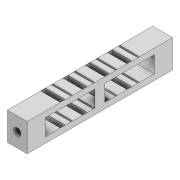
# Autodesk Inventor part: 20220727_4cell_PBME
Saved by Autodesk Inventor 2022 (Build 260153000, 153)
## iProperties
Created: 2022-07-28
Part Number: 20220727_4cell_PBME
Material: Generic
Document SubType Name: Modeling
Designer: scott
Density: 1 g/cm^3
Appearance: Default
Author: scott
Autodesk Inventor part; units mm, degrees
ref_plane "YZ Plane" through (0, 0, 0) normal (1, 0, 0) x (0, 1, 0)
ref_plane "XZ Plane" through (0, 0, 0) normal (0, 1, 0) x (-1, 0, 0)
ref_plane "XY Plane" through (0, 0, 0) normal (0, 0, 1) x (1, 0, 0)
sketch "Sketch1" plane through (0, 0, 0) normal (0, 1, 0) x (-1, 0, 0)
  line L0 (0, 0) -> (-24, 0)
  line L1 (-24, 0) -> (-24, -176.4)
  line L2 (-24, -176.4) -> (0, -176.4)
  line L3 (0, -176.4) -> (0, 0)
  dimension "d0" = 176.4
  dimension "d1" = 24
  constraints: 8 end point, 2 parallel, 1 horizontal, 1 perpendicular
  measures "d0" distance of L0.end L1.end
  measures "d1" distance of L1.end L2.end
extrude "Extrusion1" add sketch "Sketch1" along normal blind 34
sketch "Sketch2" plane through (24, 0, 0) normal (1, 0, 0) x (0, 0, -1)
  line L0 (22, 27) -> (154.4, 27)
  line L1 (154.4, 27) -> (154.4, 7)
  line L2 (154.4, 7) -> (22, 7)
  line L3 (22, 7) -> (22, 27)
  line L4 (0, 0) -> (176.4, 0) projected
  line L5 (0, 34) -> (176.4, 34) projected
  line L6 (176.4, 0) -> (176.4, 34) projected
  line L7 (0, 0) -> (0, 34) projected
  dimension "d4" = 7
  dimension "d5" = 7
  dimension "d6" = 22
  dimension "d7" = 22
  constraints: 8 end point, 2 parallel, 1 horizontal, 1 perpendicular
  measures "d4" distance between parallel lines of L4 L2
  measures "d5" distance between parallel lines of L5 L0
  measures "d6" distance between parallel lines of L6 L1
  measures "d7" distance between parallel lines of L3 L7
extrude "Extrusion2" cut sketch "Sketch2" against normal up to surface (24 mm away) contours L0 L1 L2 L3
sketch "Sketch3" plane through (0, 34, 0) normal (0, 1, 0) x (1, 0, 0)
  line L0 (0.5, 46.2) -> (23.5, 46.2)
  line L1 (23.5, 46.2) -> (23.5, 40.2)
  line L2 (23.5, 40.2) -> (0.5, 40.2)
  line L3 (0.5, 40.2) -> (0.5, 46.2)
  line L4 (0.5, 73.2) -> (23.5, 73.2)
  line L5 (23.5, 73.2) -> (23.5, 67.2)
  line L6 (23.5, 67.2) -> (0.5, 67.2)
  line L7 (0.5, 67.2) -> (0.5, 73.2)
  line L8 (0.5, 100.2) -> (23.5, 100.2)
  line L9 (23.5, 100.2) -> (23.5, 94.2)
  line L10 (23.5, 94.2) -> (0.5, 94.2)
  line L11 (0.5, 94.2) -> (0.5, 100.2)
  line L12 (0.5, 127.2) -> (23.5, 127.2)
  line L13 (23.5, 127.2) -> (23.5, 121.2)
  line L14 (23.5, 121.2) -> (0.5, 121.2)
  line L15 (0.5, 121.2) -> (0.5, 127.2)
  line L16 (0, 0) -> (24, 0) projected
  line L17 (0, 176.4) -> (0, 0) projected
  line L18 (24, 0) -> (24, 176.4) projected
  dimension "d10" = 6
  dimension "d11" = 6
  dimension "d12" = 6
  dimension "d13" = 6
  dimension "d14" = 27
  dimension "d15" = 27
  dimension "d16" = 27
  dimension "d17" = 40.2
  dimension "d18" = 0.5
  dimension "d19" = 0.5
  dimension "d20" = 0.5
  dimension "d21" = 0.5
  constraints: 32 end point, 8 parallel, 4 horizontal, 4 perpendicular, 4 point on line
  measures "d10" distance of L14.end L12.start
  measures "d11" distance of L10.end L8.start
  measures "d12" distance of L6.end L4.start
  measures "d13" distance of L2.end L0.start
  measures "d14" distance between parallel lines of L14 L10
  measures "d15" distance between parallel lines of L10 L6
  measures "d16" distance between parallel lines of L6 L2
  measures "d17" distance between parallel lines of L16 L2
  measures "d18" distance between parallel lines of L17 L3
  measures "d19" distance between parallel lines of L18 L1
  measures "d20" distance between parallel lines of L17 L7
  measures "d21" distance between parallel lines of L18 L5
extrude "Extrusion3" cut sketch "Sketch3" against normal up to surface (34 mm away)
sketch "Sketch4" plane through (0, 34, 0) normal (0, 1, 0) x (1, 0, 0)
  line L0 (0.5, 55.2) -> (23.5, 55.2)
  line L1 (23.5, 55.2) -> (23.5, 53.2)
  line L2 (23.5, 53.2) -> (0.5, 53.2)
  line L3 (0.5, 53.2) -> (0.5, 55.2)
  line L4 (0.5, 82.2) -> (23.5, 82.2)
  line L5 (23.5, 82.2) -> (23.5, 80.2)
  line L6 (23.5, 80.2) -> (0.5, 80.2)
  line L7 (0.5, 80.2) -> (0.5, 82.2)
  line L8 (0.5, 109.2) -> (23.5, 109.2)
  line L9 (23.5, 109.2) -> (23.5, 107.2)
  line L10 (23.5, 107.2) -> (0.5, 107.2)
  line L11 (0.5, 107.2) -> (0.5, 109.2)
  line L12 (0.5, 136.2) -> (23.5, 136.2)
  line L13 (23.5, 136.2) -> (23.5, 134.2)
  line L14 (23.5, 134.2) -> (0.5, 134.2)
  line L15 (0.5, 134.2) -> (0.5, 136.2)
  line L16 (0, 176.4) -> (0, 0) projected
  line L17 (24, 0) -> (24, 176.4) projected
  line L18 (0.5, 46.2) -> (23.5, 46.2) projected
  line L19 (0.5, 73.2) -> (23.5, 73.2) projected
  line L20 (0.5, 100.2) -> (23.5, 100.2) projected
  line L21 (0.5, 127.2) -> (23.5, 127.2) projected
  dimension "d24" = 0.5
  dimension "d25" = 0.5
  dimension "d26" = 2
  dimension "d27" = 2
  dimension "d28" = 2
  dimension "d29" = 2
  dimension "d30" = 7
  dimension "d31" = 7
  dimension "d32" = 7
  dimension "d33" = 7
  constraints: 32 end point, 8 parallel, 6 point on line, 4 horizontal, 4 perpendicular
  measures "d24" distance between parallel lines of L16 L3
  measures "d25" distance between parallel lines of L17 L1
  measures "d26" distance between parallel lines of L2 L0
  measures "d27" distance between parallel lines of L6 L4
  measures "d28" distance between parallel lines of L10 L8
  measures "d29" distance between parallel lines of L14 L12
  measures "d30" distance between parallel lines of L18 L2
  measures "d31" distance between parallel lines of L19 L6
  measures "d32" distance between parallel lines of L20 L10
  measures "d33" distance between parallel lines of L21 L14
extrude "Extrusion4" cut sketch "Sketch4" against normal up to surface (34 mm away)
sketch "Sketch5" plane through (0, 0, 0) normal (0, 0, 1) x (1, 0, 0)
  circle A0 centre (12, 17) radius 4.5
  line L0 (24, 0) -> (24, 34) projected
  line L1 (0, 0) -> (24, 0) projected
  dimension "d36" = 12
  dimension "d37" = 17
  dimension "d38" = 9
  constraints: 1 centre point
  measures "d36" distance from line of L0 A0.centre
  measures "d37" distance from line of L1 A0.centre
  measures "d38" diameter of A0
extrude "Extrusion5" cut sketch "Sketch5" against normal blind 12
loft "Loft1" cut section 1 edges at (7.5, 17, -12) section 2 edges at (0, 17, -22) (12, 27, -22) (24, 17, -22) (12, 7, -22)
sketch "Sketch6" plane through (24, 0, -176.4) normal (0, 0, -1) x (-1, 0, 0)
  circle A0 centre (12, 17) radius 4.5
  line L0 (24, 0) -> (24, 34) projected
  line L1 (0, 0) -> (24, 0) projected
  dimension "d45" = 12
  dimension "d46" = 17
  dimension "d47" = 9
  constraints: 1 centre point
  measures "d45" distance from line of L0 A0.centre
  measures "d46" distance from line of L1 A0.centre
  measures "d47" diameter of A0
extrude "Extrusion6" cut sketch "Sketch6" against normal blind 12
loft "Loft2" cut section 1 edges at (16.5, 17, -164.4) section 2 edges at (0, 17, -154.4) (12, 7, -154.4) (24, 17, -154.4) (12, 27, -154.4)
sketch "Sketch7" plane through (24, 0, 0) normal (1, 0, 0) x (0, 0, -1)
  line L0 (82.2, 27) -> (94.2, 27)
  line L1 (94.2, 27) -> (94.2, 7)
  line L2 (94.2, 7) -> (82.2, 7)
  line L3 (82.2, 7) -> (82.2, 27)
  line L4 (82.2, 34) -> (82.2, 27) projected
  line L5 (94.2, 34) -> (94.2, 27) projected
  line L6 (22, 27) -> (154.4, 27) projected
  line L7 (154.4, 7) -> (22, 7) projected
  point P0 (0, 0)
  dimension "d54" = 0
  dimension "d55" = 0
  dimension "d56" = 0
  dimension "d57" = 0
  constraints: 8 end point, 2 parallel, 1 horizontal, 1 perpendicular
  measures "d54" distance between parallel lines of L4 L3
  measures "d55" distance between parallel lines of L5 L1
  measures "d56" distance between parallel lines of L6 L0
  measures "d57" distance between parallel lines of L7 L2
extrude "Extrusion7" add sketch "Sketch7" against normal up to surface (24 mm away)
sketch "Sketch8" plane through (24, 7, -82.2) normal (0, 0, 1) x (1, 0, 0)
  line L0 (-23.5, 20) -> (-0.5, 20)
  line L1 (-0.5, 20) -> (-0.5, 0)
  line L2 (-0.5, 0) -> (-23.5, 0)
  line L3 (-23.5, 0) -> (-23.5, 20)
  line L4 (-24, -7) -> (-24, 27) projected
  line L5 (0, -7) -> (0, 27) projected
  line L6 (-24, 27) -> (0, 27) projected
  line L7 (-24, -7) -> (0, -7) projected
  dimension "d60" = 0.5
  dimension "d61" = 0.5
  dimension "d62" = 7
  dimension "d63" = 7
  constraints: 8 end point, 2 parallel, 1 horizontal, 1 perpendicular
  measures "d60" distance between parallel lines of L4 L3
  measures "d61" distance between parallel lines of L5 L1
  measures "d62" distance between parallel lines of L6 L0
  measures "d63" distance between parallel lines of L7 L2
extrude "Extrusion8" cut sketch "Sketch8" against normal up to surface (12 mm away) contours L0 L1 L2 L3
body "Solid1"
